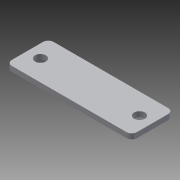
# Autodesk Inventor part: Wheel Mount Support Plate - drive wheel
Saved by Autodesk Inventor 2013 (Build 170138000, 138)
## iProperties
Created: 2013-01-25
Part Number: Wheel Mount Support Plate - drive wheel
Material: Aluminum 6061
Document SubType Name: Modeling
Designer: Moses
Mass: 15.9895 g
Surface Area: 44.7624 cm^2
Volume: 5.90017 cm^3
Density: 2.71 g/cm^3
Author: Moses
Autodesk Inventor part; units mm, degrees
ref_plane "YZ Plane" through (0, 0, 0) normal (1, 0, 0) x (0, 1, 0)
ref_plane "XZ Plane" through (0, 0, 0) normal (0, 1, 0) x (-1, 0, 0)
ref_plane "XY Plane" through (0, 0, 0) normal (0, 0, 1) x (1, 0, 0)
sketch "Sketch1" plane through (0, 0, 0) normal (0, 1, 0) x (-1, 0, 0)
  line L0 (0, 0) -> (76.2, 0)
  line L1 (76.2, 0) -> (76.2, 25.4)
  line L2 (76.2, 25.4) -> (0, 25.4)
  line L3 (0, 25.4) -> (0, 0)
  line L4 (7.9375, 12.7) -> (68.2625, 12.7) construction
  circle A0 centre (7.9375, 12.7) radius 3.302
  circle A1 centre (68.2625, 12.7) radius 3.302
  line L5 (38.1, 25.4) -> (38.1, 0) construction
  point P0 (38.1, 12.7)
  dimension "d0" = 76.2
  dimension "d1" = 6.604
  dimension "d2" = 60.325
  dimension "d3" = 25.4
  constraints: 12 end point, 4 midpoint, 2 centre point, 2 coincident, 2 parallel, 2 perpendicular, 1 equal radius, 1 horizontal
  measures "d0" distance of L1.end L2.end
  measures "d1" diameter of A0
  measures "d2" distance of L4.start L4.end
  measures "d3" distance of L2.end L0.start
extrude "Extrusion1" add sketch "Sketch1" along normal blind 3.175
fillet "Fillet1" radius 3.175 4 edges at (0, 1.5875, 25.4) (0, 1.5875, 0) (-76.2, 1.5875, 25.4) (-76.2, 1.5875, 0)
body "Solid1"
